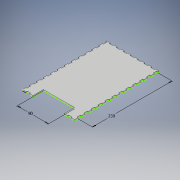
# Autodesk Inventor part: base_caja
Saved by Autodesk Inventor 2019 (Build 230136000, 136)
## iProperties
Created: 2018-05-30
Part Number: base_caja
Material: Generic
Document SubType Name: Modeling
Designer: seba
Density: 1 g/cm^3
Appearance: Default
Author: seba
Autodesk Inventor part; units mm, degrees
ref_plane "YZ Plane" through (0, 0, 0) normal (1, 0, 0) x (0, 1, 0)
ref_plane "XZ Plane" through (0, 0, 0) normal (0, 1, 0) x (-1, 0, 0)
ref_plane "XY Plane" through (0, 0, 0) normal (0, 0, 1) x (1, 0, 0)
sketch "Sketch1" plane through (0, 0, 0) normal (0, 1, 0) x (-1, 0, 0)
  line L0 (0, -10) -> (-3, -10)
  line L1 (-3, -10) -> (-3, -20)
  line L2 (-3, -20) -> (0, -20)
  line L3 (0, -30) -> (-3, -30)
  line L4 (-3, -30) -> (-3, -40)
  line L5 (-3, -40) -> (0, -40)
  line L6 (0, -40) -> (0, -50)
  line L7 (0, -50) -> (-3, -50)
  line L8 (-3, -50) -> (-3, -60)
  line L9 (-3, -60) -> (0, -60)
  line L10 (0, -60) -> (0, -70)
  line L11 (0, -70) -> (-3, -70)
  line L12 (-3, -70) -> (-3, -80)
  line L13 (-3, -80) -> (0, -80)
  line L14 (0, -80) -> (0, -90)
  line L15 (0, -90) -> (-3, -90)
  line L16 (-3, -90) -> (-3, -100)
  line L17 (-3, -100) -> (0, -100)
  line L18 (0, -100) -> (0, -110)
  line L19 (0, -110) -> (-3, -110)
  line L20 (-3, -110) -> (-3, -120)
  line L21 (-3, -120) -> (0, -120)
  line L22 (0, -120) -> (0, -130)
  line L23 (0, -130) -> (-3, -130)
  line L24 (-3, -130) -> (-3, -140)
  line L25 (-3, -140) -> (0, -140)
  line L26 (0, -140) -> (0, -150)
  line L27 (0, -150) -> (-3, -150)
  line L28 (-3, -150) -> (-3, -160)
  line L29 (-3, -160) -> (0, -160)
  line L30 (0, -160) -> (0, -170)
  line L31 (0, -170) -> (-3, -170)
  line L32 (-3, -170) -> (-3, -180)
  line L33 (-3, -180) -> (0, -180)
  line L34 (0, -180) -> (0, -190)
  line L35 (0, -190) -> (-3, -190)
  line L36 (-3, -190) -> (-3, -200)
  line L37 (-3, -200) -> (0, -200)
  line L38 (0, -200) -> (0, -210)
  line L39 (0, -210) -> (-3, -210)
  line L40 (-3, -210) -> (-3, -220)
  line L41 (-3, -220) -> (0, -220)
  line L42 (0, -220) -> (0, -230)
  line L43 (0, -230) -> (-3, -230)
  line L44 (-3, -230) -> (-3, -240)
  line L45 (-3, -240) -> (0, -240)
  line L46 (0, -240) -> (0, -243)
  line L47 (0, -243) -> (-10, -243)
  line L48 (-10, -243) -> (-10, -240)
  line L49 (-10, -240) -> (-20, -240)
  line L50 (-20, -240) -> (-20, -243)
  line L51 (-20, -243) -> (-30, -243)
  line L52 (-30, -243) -> (-30, -240)
  line L53 (-30, -240) -> (-40, -240)
  line L54 (-40, -240) -> (-40, -243)
  line L55 (-40, -243) -> (-50, -243)
  line L56 (-50, -243) -> (-50, -240)
  line L57 (-50, -240) -> (-60, -240)
  line L58 (-60, -240) -> (-60, -243)
  line L59 (-60, -243) -> (-70, -243)
  line L60 (-70, -243) -> (-70, -240)
  line L61 (-70, -240) -> (-80, -240)
  line L62 (-80, -240) -> (-80, -243)
  line L63 (-80, -243) -> (-90, -243)
  line L64 (-90, -243) -> (-90, -240)
  line L65 (-90, -240) -> (-100, -240)
  line L66 (-100, -240) -> (-100, -243)
  line L67 (-100, -243) -> (-110, -243)
  line L68 (-110, -243) -> (-110, -240)
  line L69 (-110, -240) -> (-120, -240)
  line L70 (-120, -240) -> (-120, -243)
  line L71 (-120, -243) -> (-130, -243)
  line L72 (-130, -243) -> (-130, -240)
  line L73 (-130, -240) -> (-140, -240)
  line L74 (-140, -240) -> (-140, -243)
  line L75 (-140, -243) -> (-150, -243)
  line L76 (-150, -243) -> (-150, -240)
  line L77 (-150, -240) -> (-147, -240)
  line L78 (-147, -240) -> (-147, -230)
  line L79 (-147, -230) -> (-150, -230)
  line L80 (-150, -230) -> (-150, -220)
  line L81 (-150, -220) -> (-147, -220)
  line L82 (-147, -220) -> (-147, -210)
  line L83 (-147, -210) -> (-150, -210)
  line L84 (-150, -210) -> (-150, -200)
  line L85 (-150, -200) -> (-147, -200)
  line L86 (-147, -200) -> (-147, -190)
  line L87 (-147, -190) -> (-150, -190)
  line L88 (-150, -190) -> (-150, -180)
  line L89 (-150, -180) -> (-147, -180)
  line L90 (-147, -180) -> (-147, -170)
  line L91 (-147, -170) -> (-150, -170)
  line L92 (-150, -170) -> (-150, -160)
  line L93 (-150, -160) -> (-147, -160)
  line L94 (-147, -160) -> (-147, -150)
  line L95 (-147, -150) -> (-150, -150)
  line L96 (-150, -150) -> (-150, -140)
  line L97 (-150, -140) -> (-147, -140)
  line L98 (-147, -140) -> (-147, -130)
  line L99 (-147, -130) -> (-150, -130)
  line L100 (-150, -130) -> (-150, -120)
  line L101 (-150, -120) -> (-147, -120)
  line L102 (-147, -120) -> (-147, -110)
  line L103 (-147, -110) -> (-150, -110)
  line L104 (-150, -110) -> (-150, -100)
  line L105 (-150, -100) -> (-147, -100)
  line L106 (-147, -100) -> (-147, -90)
  line L107 (-147, -90) -> (-150, -90)
  line L108 (-150, -90) -> (-150, -80)
  line L109 (-150, -80) -> (-147, -80)
  line L110 (-147, -80) -> (-147, -70)
  line L111 (-147, -70) -> (-150, -70)
  line L112 (-150, -70) -> (-150, -60)
  line L113 (-150, -60) -> (-147, -60)
  line L114 (-147, -60) -> (-147, -50)
  line L115 (-147, -50) -> (-150, -50)
  line L116 (-150, -50) -> (-150, -40)
  line L117 (-150, -40) -> (-147, -40)
  line L118 (-147, -40) -> (-147, -30)
  line L119 (-147, -30) -> (-150, -30)
  line L120 (-150, -30) -> (-150, -20)
  line L121 (-150, -20) -> (-147, -20)
  line L122 (-147, -20) -> (-147, -10)
  line L123 (-147, -10) -> (-150, -10)
  line L124 (-150, -10) -> (-150, 0)
  line L125 (-150, 0) -> (-140, 0)
  line L126 (-140, 0) -> (-140, -3)
  line L127 (-140, -3) -> (-130, -3)
  line L128 (-130, -3) -> (-130, 0)
  line L129 (-130, 0) -> (-120, 0)
  line L130 (-120, 0) -> (-120, -5)
  line L131 (-120, 0) -> (-120, -5)
  line L132 (-120, -5) -> (-120, -10)
  line L133 (-120, -20) -> (-120, -30)
  line L134 (-10, 0) -> (-10, -3)
  line L135 (-10, -3) -> (-20, -3)
  line L136 (-20, -3) -> (-20, 0)
  line L137 (-20, 0) -> (-30, 0)
  line L138 (-30, 0) -> (-30, -10)
  line L139 (-30, -20) -> (-30, -30)
  line L140 (-30, -30) -> (-120, -30)
  line L141 (0, -20) -> (0, -30)
  line L142 (0, -10) -> (0, 0)
  line L143 (0, 0) -> (-10, 0)
  line L144 (-120, -20) -> (-120, -5)
  line L145 (-30, -7.5) -> (-30, -20)
  dimension "d165" = 230
  dimension "d200" = 90
  constraints: 292 end point, 93 point on line, 80 perpendicular, 13 horizontal, 5 vertical, 1 collinear
  measures "d165" distance of L123.end L76.end
  measures "d200" distance of L139.end L133.end
extrude "Extrusion1" add sketch "Sketch1" along normal blind 3
sketch "Sketch2" plane through (0, 3, 0) normal (0, 1, 0) x (1, 0, 0)
  point P0 (0, 0)
body "Solid1"
